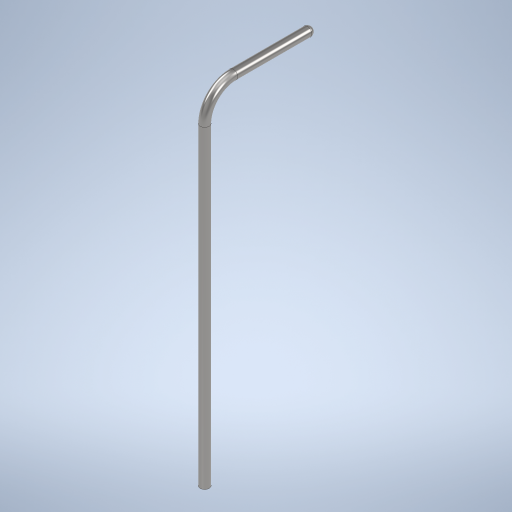
# Autodesk Inventor part: Pitot Tube
Saved by Autodesk Inventor 2023 (Build 270158000, 158)
## iProperties
Created: 2022-09-15
Part Number: Pitot Tube
Material: Stainless Steel
Document SubType Name: Modeling
Designer: earls
Density: 8 g/cm^3
Appearance: Semi-Polished
Author: earls
Autodesk Inventor part; units mm, degrees
ref_plane "YZ Plane" through (0, 0, 0) normal (1, 0, 0) x (0, 1, 0)
ref_plane "XZ Plane" through (0, 0, 0) normal (0, 1, 0) x (-1, 0, 0)
ref_plane "XY Plane" through (0, 0, 0) normal (0, 0, 1) x (1, 0, 0)
sketch "Sketch1" plane through (0, 0, 0) normal (0, 1, 0) x (-1, 0, 0)
  circle A0 centre (0, 0) radius 3.9688
  circle A1 centre (0, 0) radius 2.9688
  dimension "d0" = 7.9375
  dimension "d4" = 1
  constraints: 2 centre point, 1 coincident
  measures "d0" diameter of A0
  measures "d4" radial gap between concentric circles of A0 A1
sketch "Sketch2" plane through (0, 0, 0) normal (1, 0, 0) x (0, 1, 0)
  line L0 (0, 0) -> (275, 0)
  line L1 (300, -25) -> (300, -90)
  arc A0 (300, -25) -> (275, 0) centre (275, -25) ccw
  point P0 (300, 0)
  dimension "d1" = 300
  dimension "d2" = 90
  dimension "d3" = 25
  constraints: 4 end point, 2 point on circle, 2 point on line, 2 tangent, 1 centre point, 1 horizontal, 1 perpendicular
  measures "d1" distance of L0.start point (300, 0)
  measures "d2" distance of point (300, 0) L1.end
  measures "d3" radius of A0
sweep "Sweep1" add profiles "Sketch1" path "Sketch2"
sketch "Sketch3" plane through (0, 0, 0) normal (1, 0, 0) x (0, 1, 0)
  line L0 (296.0312, -90) -> (303.9688, -90) projected
  arc A0 (300.25, -93.9609) -> (299.75, -93.9609) centre (300, -90) ccw
  line L1 (300, -90) -> (300, -93.9688)
  line L2 (300.25, -90) -> (300.25, -93.9609)
  line L3 (299.75, -90) -> (299.75, -93.9609)
  point P0 (0, 0)
  point P1 (300.25, -96.7948)
  point P2 (299.75, -96.7948)
  dimension "d7" = 0.25
  constraints: 6 end point, 3 point on circle, 2 symmetric about line, 1 centre point, 1 midpoint, 1 parallel, 1 vertical
  measures "d7" distance between parallel lines of L1 L2
revolve "Revolution1" add sketch "Sketch3" angle 360 about axis through (0, 300, -90) along (0, 0, -1) contours A0 L2 L0
body "Solid1"
